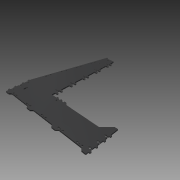
# Autodesk Inventor part: brace_right
Saved by Autodesk Inventor 2014 (Build 180170000, 170)
## iProperties
Created: 2013-12-03
Part Number: brace_right
Material: Generic
Document SubType Name: Modeling
Designer: buben
Density: 1 g/cm^3
Appearance: Anodized - Dark Gray
Author: buben
Subject: Laser Cutted
Autodesk Inventor part; units mm, degrees
ref_plane "YZ Plane" through (0, 0, 0) normal (1, 0, 0) x (0, 1, 0)
ref_plane "XZ Plane" through (0, 0, 0) normal (0, 1, 0) x (-1, 0, 0)
ref_plane "XY Plane" through (0, 0, 0) normal (0, 0, 1) x (1, 0, 0)
sketch "Sketch1" plane through (0, 0, 0) normal (0, 0, 1) x (1, 0, 0)
  line L0 (0, 0) -> (489, 0)
  line L1 (489, 0) -> (489, 150)
  line L2 (0, 0) -> (0, 120)
  line L3 (0, 120) -> (106.25, 518.5)
  line L4 (106.25, 518.5) -> (156.25, 518.5)
  line L5 (156.25, 518.5) -> (156.25, 113.5)
  line L6 (489, 150) -> (474, 150)
  line L7 (474, 150) -> (434, 110)
  line L8 (434, 110) -> (253.25, 110)
  line L9 (253.25, 110) -> (243.25, 120)
  line L10 (243.25, 120) -> (233.25, 120)
  line L11 (233.25, 120) -> (233.25, 113.5)
  line L12 (233.25, 113.5) -> (156.25, 113.5)
  point P0 (244.5, 0)
  dimension "d0" = 489
  dimension "d2" = 120
  dimension "d3" = 45
  dimension "d5" = 6.5
  dimension "d6" = 77
  dimension "d7" = 15
  dimension "d8" = 10
  dimension "d9" = 50
  dimension "d10" = 518.5
  dimension "d13" = 10
  dimension "d261" = 156.25
  dimension "d289" = 150
  dimension "d290" = 40
  constraints: 26 end point, 7 perpendicular, 3 parallel, 1 horizontal, 1 midpoint
  measures "d0" distance of L0.start L0.end
  measures "d2" distance of L0.start L2.end
  measures "d3" angle of L6 L7
  measures "d5" distance of L10.end L11.end
  measures "d6" distance of L11.end L5.end
  measures "d7" distance of L1.end L6.end
  measures "d8" distance of L9.end L10.end
  measures "d9" distance of L3.end L4.end
  measures "d10" distance between parallel lines of L0 L4
  measures "d13" distance between parallel lines of L8 L10
  measures "d261" distance between parallel lines of L2 L5
  measures "d289" distance of L0.end L1.end
  measures "d290" distance between parallel lines of L6 L8
extrude "Extrusion1" add sketch "Sketch1" along normal blind 6.5
sketch "Sketch2" plane through (0, 0, 6.5) normal (0, 0, 1) x (1, 0, 0)
  line L0 (0, 0) -> (489, 0) projected
  line L1 (489, 0) -> (489, 150) projected
  line L2 (253.25, 110) -> (243.25, 120) projected
  line L3 (489, 20.75) -> (489, 16.25)
  line L4 (472.7, 16.25) -> (472.7, 20.75)
  line L5 (476.7, 23.25) -> (484, 23.25)
  line L6 (484, 13.75) -> (476.7, 13.75)
  line L7 (472.7, 20.75) -> (476.7, 20.75)
  line L8 (484, 20.75) -> (489, 20.75)
  line L9 (489, 16.25) -> (484, 16.25)
  line L10 (476.7, 16.25) -> (472.7, 16.25)
  line L11 (476.7, 13.75) -> (476.7, 16.25)
  line L12 (476.7, 20.75) -> (476.7, 23.25)
  line L13 (484, 23.25) -> (484, 20.75)
  line L14 (484, 16.25) -> (484, 13.75)
  line L15 (489, 98.75) -> (489, 94.25)
  line L16 (472.7, 94.25) -> (472.7, 98.75)
  line L17 (476.7, 101.25) -> (484, 101.25)
  line L18 (484, 91.75) -> (476.7, 91.75)
  line L19 (472.7, 98.75) -> (476.7, 98.75)
  line L20 (484, 98.75) -> (489, 98.75)
  line L21 (489, 94.25) -> (484, 94.25)
  line L22 (476.7, 94.25) -> (472.7, 94.25)
  line L23 (476.7, 91.75) -> (476.7, 94.25)
  line L24 (476.7, 98.75) -> (476.7, 101.25)
  line L25 (484, 101.25) -> (484, 98.75)
  line L26 (484, 94.25) -> (484, 91.75)
  line L27 (489, 59.75) -> (489, 55.25)
  line L28 (472.7, 55.25) -> (472.7, 59.75)
  line L29 (476.7, 62.25) -> (484, 62.25)
  line L30 (484, 52.75) -> (476.7, 52.75)
  line L31 (472.7, 59.75) -> (476.7, 59.75)
  line L32 (484, 59.75) -> (489, 59.75)
  line L33 (489, 55.25) -> (484, 55.25)
  line L34 (476.7, 55.25) -> (472.7, 55.25)
  line L35 (476.7, 52.75) -> (476.7, 55.25)
  line L36 (476.7, 59.75) -> (476.7, 62.25)
  line L37 (484, 62.25) -> (484, 59.75)
  line L38 (484, 55.25) -> (484, 52.75)
  line L39 (244.5, 0) -> (244.5, 118.75) construction
  line L40 (0, 20.75) -> (0, 16.25)
  line L41 (16.3, 16.25) -> (16.3, 20.75)
  line L42 (12.3, 23.25) -> (5, 23.25)
  line L43 (5, 13.75) -> (12.3, 13.75)
  line L44 (16.3, 20.75) -> (12.3, 20.75)
  line L45 (5, 20.75) -> (0, 20.75)
  line L46 (0, 16.25) -> (5, 16.25)
  line L47 (12.3, 16.25) -> (16.3, 16.25)
  line L48 (12.3, 13.75) -> (12.3, 16.25)
  line L49 (12.3, 20.75) -> (12.3, 23.25)
  line L50 (5, 23.25) -> (5, 20.75)
  line L51 (5, 16.25) -> (5, 13.75)
  line L52 (16.3, 98.75) -> (12.3, 98.75)
  line L53 (16.3, 94.25) -> (16.3, 98.75)
  line L54 (12.3, 94.25) -> (16.3, 94.25)
  line L55 (12.3, 98.75) -> (12.3, 101.25)
  line L56 (12.3, 91.75) -> (12.3, 94.25)
  line L57 (12.3, 101.25) -> (5, 101.25)
  line L58 (5, 94.25) -> (5, 91.75)
  line L59 (5, 91.75) -> (12.3, 91.75)
  line L60 (5, 98.75) -> (0, 98.75)
  line L61 (0, 98.75) -> (0, 94.25)
  line L62 (0, 94.25) -> (5, 94.25)
  line L63 (5, 101.25) -> (5, 98.75)
  line L64 (12.3, 59.75) -> (12.3, 62.25)
  line L65 (16.3, 59.75) -> (12.3, 59.75)
  line L66 (16.3, 55.25) -> (16.3, 59.75)
  line L67 (12.3, 55.25) -> (16.3, 55.25)
  line L68 (12.3, 52.75) -> (12.3, 55.25)
  line L69 (12.3, 62.25) -> (5, 62.25)
  line L70 (5, 52.75) -> (12.3, 52.75)
  line L71 (5, 55.25) -> (5, 52.75)
  line L72 (5, 62.25) -> (5, 59.75)
  line L73 (0, 55.25) -> (5, 55.25)
  line L74 (5, 59.75) -> (0, 59.75)
  line L75 (0, 59.75) -> (0, 55.25)
  point P0 (472.7, 18.5)
  point P1 (480.35, 23.25)
  point P2 (472.7, 96.5)
  point P3 (480.35, 101.25)
  point P4 (472.7, 57.5)
  point P5 (480.35, 62.25)
  point P6 (16.3, 18.5)
  point P7 (8.65, 23.25)
  point P8 (16.3, 96.5)
  point P9 (8.65, 101.25)
  point P10 (16.3, 57.5)
  point P11 (8.65, 62.25)
  dimension "d16" = 4.5
  dimension "d17" = 2.5
  dimension "d18" = 2.5
  dimension "d19" = 4
  dimension "d20" = 7.3
  dimension "d21" = 5
  dimension "d23" = 4.5
  dimension "d24" = 2.5
  dimension "d25" = 2.5
  dimension "d26" = 4
  dimension "d27" = 7.3
  dimension "d28" = 5
  dimension "d30" = 4.5
  dimension "d31" = 2.5
  dimension "d32" = 2.5
  dimension "d33" = 4
  dimension "d34" = 7.3
  dimension "d35" = 5
  dimension "d40" = 18.5
  dimension "d41" = 39
  dimension "d42" = 39
  constraints: 146 end point, 42 symmetric about line, 30 parallel, 15 collinear, 13 perpendicular, 9 horizontal, 7 midpoint, 1 point on line
  measures "d16" distance of L4.start L4.end
  measures "d17" distance of L7.end L5.start
  measures "d18" distance of L6.end L10.start
  measures "d19" distance of L10.start L4.start
  measures "d20" distance of L6.start L6.end
  measures "d21" distance of L3.end L9.end
  measures "d23" distance of L16.start L19.start
  measures "d24" distance of L19.end L24.end
  measures "d25" distance of L23.start L22.start
  measures "d26" distance of L22.start L16.start
  measures "d27" distance of L26.end L23.start
  measures "d28" distance of L15.end L26.start
  measures "d30" distance of L28.start L31.start
  measures "d31" distance of L36.start L36.end
  measures "d32" distance of L35.start L34.start
  measures "d33" distance of L34.start L28.start
  measures "d34" distance of L30.start L35.start
  measures "d35" distance of L33.start L38.start
  measures "d40" distance from line of L0 point (472.7, 18.5)
  measures "d41" distance of point (472.7, 57.5) point (472.7, 18.5)
  measures "d42" distance of point (472.7, 57.5) point (472.7, 96.5)
extrude "Extrusion2" cut sketch "Sketch2" against normal through all
sketch "Sketch4" plane through (0, 0, 6.5) normal (0, 0, 1) x (1, 0, 0)
  line L0 (0, 16.25) -> (0, 0) projected
  line L1 (489, 0) -> (489, 16.25) projected
  line L2 (472.7, 16.25) -> (472.7, 20.75) projected
  line L3 (489, 20.75) -> (489, 55.25) projected
  line L4 (472.7, 55.25) -> (472.7, 59.75) projected
  line L5 (489, 59.75) -> (489, 94.25) projected
  line L6 (472.7, 94.25) -> (472.7, 98.75) projected
  line L7 (489, 98.75) -> (489, 150) projected
  line L8 (0, 120) -> (0, 98.75) projected
  line L9 (0, 94.25) -> (0, 59.75) projected
  line L10 (0, 55.25) -> (0, 20.75) projected
  line L11 (0, 112) -> (-4.5, 112)
  line L12 (-6.5, 110) -> (-6.5, 106)
  line L13 (-4.5, 104) -> (0, 104)
  line L14 (0, 104) -> (0, 112)
  line L15 (0, 81) -> (-4.5, 81)
  line L16 (-6.5, 79) -> (-6.5, 75)
  line L17 (-4.5, 73) -> (0, 73)
  line L18 (0, 73) -> (0, 81)
  line L19 (0, 42) -> (-4.5, 42)
  line L20 (-6.5, 40) -> (-6.5, 36)
  line L21 (-4.5, 34) -> (0, 34)
  line L22 (0, 34) -> (0, 42)
  line L23 (0, 11) -> (-4.5, 11)
  line L24 (-6.5, 9) -> (-6.5, 5)
  line L25 (-4.5, 3) -> (0, 3)
  line L26 (0, 3) -> (0, 11)
  line L27 (489, 112) -> (493.5, 112)
  line L28 (495.5, 110) -> (495.5, 106)
  line L29 (493.5, 104) -> (489, 104)
  line L30 (489, 104) -> (489, 112)
  line L31 (489, 81) -> (493.5, 81)
  line L32 (495.5, 79) -> (495.5, 75)
  line L33 (493.5, 73) -> (489, 73)
  line L34 (489, 73) -> (489, 81)
  line L35 (489, 42) -> (493.5, 42)
  line L36 (495.5, 40) -> (495.5, 36)
  line L37 (493.5, 34) -> (489, 34)
  line L38 (489, 34) -> (489, 42)
  line L39 (489, 11) -> (493.5, 11)
  line L40 (495.5, 9) -> (495.5, 5)
  line L41 (493.5, 3) -> (489, 3)
  line L42 (489, 3) -> (489, 11)
  arc A0 (-6.5, 5) -> (-4.5, 3) centre (-4.5, 5) ccw
  arc A1 (-4.5, 11) -> (-6.5, 9) centre (-4.5, 9) ccw
  arc A2 (-6.5, 36) -> (-4.5, 34) centre (-4.5, 36) ccw
  arc A3 (-4.5, 42) -> (-6.5, 40) centre (-4.5, 40) ccw
  arc A4 (-6.5, 75) -> (-4.5, 73) centre (-4.5, 75) ccw
  arc A5 (-4.5, 81) -> (-6.5, 79) centre (-4.5, 79) ccw
  arc A6 (-6.5, 106) -> (-4.5, 104) centre (-4.5, 106) ccw
  arc A7 (-4.5, 112) -> (-6.5, 110) centre (-4.5, 110) ccw
  arc A8 (495.5, 110) -> (493.5, 112) centre (493.5, 110) ccw
  arc A9 (493.5, 104) -> (495.5, 106) centre (493.5, 106) ccw
  arc A10 (495.5, 79) -> (493.5, 81) centre (493.5, 79) ccw
  arc A11 (493.5, 73) -> (495.5, 75) centre (493.5, 75) ccw
  arc A12 (495.5, 40) -> (493.5, 42) centre (493.5, 40) ccw
  arc A13 (493.5, 34) -> (495.5, 36) centre (493.5, 36) ccw
  arc A14 (495.5, 9) -> (493.5, 11) centre (493.5, 9) ccw
  arc A15 (493.5, 3) -> (495.5, 5) centre (493.5, 5) ccw
  line L43 (489, 20.75) -> (489, 55.25) projected
  point P0 (472.7, 96.5)
  point P1 (472.7, 57.5)
  point P2 (472.7, 18.5)
  point P3 (495.5, 77)
  point P4 (489, 77)
  point P5 (495.5, 38)
  point P6 (489, 38)
  dimension "d81" = 2
  dimension "d82" = 8
  dimension "d83" = 8
  dimension "d84" = 8
  dimension "d85" = 8
  dimension "d86" = 7.5
  dimension "d87" = 7.5
  dimension "d88" = 6.5
  dimension "d89" = 6.5
  constraints: 64 end point, 32 point on circle, 32 tangent, 16 centre point, 16 parallel, 15 equal radius, 14 collinear, 8 horizontal, 8 perpendicular, 8 point on line, 7 midpoint, 2 horizontal alignment
  measures "d81" radius of A0
  measures "d82" distance between parallel lines of L29 L27
  measures "d83" distance between parallel lines of L33 L31
  measures "d84" distance between parallel lines of L37 L35
  measures "d85" distance between parallel lines of L41 L39
  measures "d86" distance from line of point (472.7, 96.5) L29
  measures "d87" distance from line of point (472.7, 18.5) L39
  measures "d88" distance between parallel lines of L7 L28
  measures "d89" distance between parallel lines of L8 L12
extrude "Extrusion4" add sketch "Sketch4" against normal blind 6.5
sketch "Sketch5" plane through (0, 0, 6.5) normal (0, 0, 1) x (1, 0, 0)
  line L0 (233.25, 120) -> (233.25, 113.5) projected
  line L1 (233.25, 113.5) -> (156.25, 113.5) projected
  line L2 (201.5, 113.5) -> (206, 113.5)
  line L3 (206, 97.2) -> (201.5, 97.2)
  line L4 (208.5, 108.5) -> (208.5, 101.2)
  line L5 (199, 101.2) -> (199, 108.5)
  line L6 (206, 113.5) -> (206, 108.5)
  line L7 (206, 101.2) -> (206, 97.2)
  line L8 (201.5, 97.2) -> (201.5, 101.2)
  line L9 (201.5, 108.5) -> (201.5, 113.5)
  line L10 (199, 108.5) -> (201.5, 108.5)
  line L11 (206, 108.5) -> (208.5, 108.5)
  line L12 (208.5, 101.2) -> (206, 101.2)
  line L13 (201.5, 101.2) -> (199, 101.2)
  point P0 (203.75, 97.2)
  dimension "d92" = 4.5
  dimension "d93" = 2.5
  dimension "d94" = 2.5
  dimension "d95" = 5
  dimension "d96" = 7.3
  dimension "d97" = 4
  dimension "d98" = 29.5
  constraints: 24 end point, 10 parallel, 5 collinear, 4 perpendicular, 3 horizontal, 1 midpoint
  measures "d92" distance of L3.start L3.end
  measures "d93" distance of L8.end L5.start
  measures "d94" distance of L4.end L7.start
  measures "d95" distance of L2.end L6.end
  measures "d96" distance of L4.start L4.end
  measures "d97" distance of L7.start L3.start
  measures "d98" distance from line of L0 point (203.75, 97.2)
extrude "Extrusion5" cut sketch "Sketch5" against normal through all
sketch "Sketch6" plane through (0, 0, 6.5) normal (0, 0, 1) x (1, 0, 0)
  line L0 (206, 97.2) -> (201.5, 97.2) projected
  line L1 (201.5, 113.5) -> (156.25, 113.5) projected
  line L2 (233.25, 113.5) -> (206, 113.5) projected
  line L3 (188.25, 113.5) -> (196.25, 113.5)
  line L4 (196.25, 113.5) -> (196.25, 118)
  line L5 (194.25, 120) -> (190.25, 120)
  line L6 (188.25, 118) -> (188.25, 113.5)
  line L7 (211.25, 113.5) -> (219.25, 113.5)
  line L8 (219.25, 113.5) -> (219.25, 118)
  line L9 (217.25, 120) -> (213.25, 120)
  line L10 (211.25, 118) -> (211.25, 113.5)
  arc A0 (190.25, 120) -> (188.25, 118) centre (190.25, 118) ccw
  arc A1 (196.25, 118) -> (194.25, 120) centre (194.25, 118) ccw
  arc A2 (213.25, 120) -> (211.25, 118) centre (213.25, 118) ccw
  arc A3 (219.25, 118) -> (217.25, 120) centre (217.25, 118) ccw
  point P0 (203.75, 97.2)
  dimension "d101" = 2
  dimension "d102" = 15
  dimension "d103" = 8
  dimension "d104" = 8
  dimension "d105" = 7.5
  dimension "d106" = 6.5
  constraints: 16 end point, 8 point on circle, 8 tangent, 4 centre point, 4 parallel, 3 equal radius, 2 horizontal, 2 perpendicular, 2 point on line, 1 collinear, 1 midpoint
  measures "d101" radius of A0
  measures "d102" distance between parallel lines of L4 L10
  measures "d103" distance between parallel lines of L6 L4
  measures "d104" distance between parallel lines of L8 L10
  measures "d105" distance from line of point (203.75, 97.2) L4
  measures "d106" distance between parallel lines of L1 L5
extrude "Extrusion6" add sketch "Sketch6" against normal blind 6.5
sketch "Sketch7" plane through (0, 0, 6.5) normal (0, 0, 1) x (1, 0, 0)
  line L0 (156.25, 113.5) -> (156.25, 518.5) projected
  line L1 (156.25, 518.5) -> (106.25, 518.5) projected
  line L2 (121.25, 451) -> (113.25, 451)
  line L3 (113.25, 451) -> (113.25, 444.5)
  line L4 (113.25, 444.5) -> (121.25, 444.5)
  line L5 (121.25, 444.5) -> (121.25, 451)
  circle A0 centre (128.75, 447.75) radius 2.25
  point P0 (121.25, 447.75)
  dimension "d109" = 6.5
  dimension "d110" = 8
  dimension "d118" = 7.5
  dimension "d119" = 27.5
  dimension "d121" = 4.5
  dimension "d288" = 74
  constraints: 8 end point, 2 parallel, 1 centre point, 1 horizontal, 1 horizontal alignment, 1 midpoint, 1 perpendicular
  measures "d109" distance of L2.end L3.end
  measures "d110" distance of L2.start L2.end
  measures "d118" distance from line of A0.centre L5
  measures "d119" distance from line of L0 A0.centre
  measures "d121" diameter of A0
  measures "d288" distance between parallel lines of L4 L1
extrude "Extrusion8" cut sketch "Sketch7" against normal through all
sketch "Sketch8" plane through (0, 0, 6.5) normal (0, 0, 1) x (1, 0, 0)
  line L0 (156.25, 518.5) -> (112.25, 518.5)
  line L1 (112.25, 518.5) -> (112.25, 512)
  line L2 (112.25, 512) -> (156.25, 512)
  line L3 (156.25, 512) -> (156.25, 518.5)
  point P0 (106.25, 518.5)
  dimension "d124" = 6
  dimension "d125" = 6.5
  constraints: 8 end point, 2 parallel, 1 horizontal, 1 perpendicular
  measures "d124" distance from line of point (106.25, 518.5) L1
  measures "d125" distance of L0.end L1.end
extrude "Extrusion9" cut sketch "Sketch8" against normal through all
sketch "Sketch9" plane through (0, 0, 6.5) normal (0, 0, 1) x (1, 0, 0)
  line L0 (156.25, 113.5) -> (156.25, 512) projected
  line L1 (156.25, 470.75) -> (156.25, 466.25)
  line L2 (139.95, 466.25) -> (139.95, 470.75)
  line L3 (143.95, 473.25) -> (151.25, 473.25)
  line L4 (151.25, 463.75) -> (143.95, 463.75)
  line L5 (151.25, 473.25) -> (151.25, 470.75)
  line L6 (151.25, 466.25) -> (151.25, 463.75)
  line L7 (143.95, 463.75) -> (143.95, 466.25)
  line L8 (143.95, 470.75) -> (143.95, 473.25)
  line L9 (139.95, 470.75) -> (143.95, 470.75)
  line L10 (151.25, 470.75) -> (156.25, 470.75)
  line L11 (156.25, 466.25) -> (151.25, 466.25)
  line L12 (143.95, 466.25) -> (139.95, 466.25)
  line L13 (156.25, 390.75) -> (156.25, 386.25)
  line L14 (139.95, 386.25) -> (139.95, 390.75)
  line L15 (143.95, 393.25) -> (151.25, 393.25)
  line L16 (151.25, 383.75) -> (143.95, 383.75)
  line L17 (151.25, 393.25) -> (151.25, 390.75)
  line L18 (151.25, 386.25) -> (151.25, 383.75)
  line L19 (143.95, 383.75) -> (143.95, 386.25)
  line L20 (143.95, 390.75) -> (143.95, 393.25)
  line L21 (139.95, 390.75) -> (143.95, 390.75)
  line L22 (151.25, 390.75) -> (156.25, 390.75)
  line L23 (156.25, 386.25) -> (151.25, 386.25)
  line L24 (143.95, 386.25) -> (139.95, 386.25)
  line L25 (156.25, 310.75) -> (156.25, 306.25)
  line L26 (139.95, 306.25) -> (139.95, 310.75)
  line L27 (143.95, 313.25) -> (151.25, 313.25)
  line L28 (151.25, 303.75) -> (143.95, 303.75)
  line L29 (151.25, 313.25) -> (151.25, 310.75)
  line L30 (151.25, 306.25) -> (151.25, 303.75)
  line L31 (143.95, 303.75) -> (143.95, 306.25)
  line L32 (143.95, 310.75) -> (143.95, 313.25)
  line L33 (139.95, 310.75) -> (143.95, 310.75)
  line L34 (151.25, 310.75) -> (156.25, 310.75)
  line L35 (156.25, 306.25) -> (151.25, 306.25)
  line L36 (143.95, 306.25) -> (139.95, 306.25)
  line L37 (156.25, 230.75) -> (156.25, 226.25)
  line L38 (139.95, 226.25) -> (139.95, 230.75)
  line L39 (143.95, 233.25) -> (151.25, 233.25)
  line L40 (151.25, 223.75) -> (143.95, 223.75)
  line L41 (151.25, 233.25) -> (151.25, 230.75)
  line L42 (151.25, 226.25) -> (151.25, 223.75)
  line L43 (143.95, 223.75) -> (143.95, 226.25)
  line L44 (143.95, 230.75) -> (143.95, 233.25)
  line L45 (139.95, 230.75) -> (143.95, 230.75)
  line L46 (151.25, 230.75) -> (156.25, 230.75)
  line L47 (156.25, 226.25) -> (151.25, 226.25)
  line L48 (143.95, 226.25) -> (139.95, 226.25)
  line L49 (156.25, 150.75) -> (156.25, 146.25)
  line L50 (139.95, 146.25) -> (139.95, 150.75)
  line L51 (143.95, 153.25) -> (151.25, 153.25)
  line L52 (151.25, 143.75) -> (143.95, 143.75)
  line L53 (151.25, 153.25) -> (151.25, 150.75)
  line L54 (151.25, 146.25) -> (151.25, 143.75)
  line L55 (143.95, 143.75) -> (143.95, 146.25)
  line L56 (143.95, 150.75) -> (143.95, 153.25)
  line L57 (139.95, 150.75) -> (143.95, 150.75)
  line L58 (151.25, 150.75) -> (156.25, 150.75)
  line L59 (156.25, 146.25) -> (151.25, 146.25)
  line L60 (143.95, 146.25) -> (139.95, 146.25)
  line L61 (112.25, 518.5) -> (106.25, 518.5) projected
  point P0 (139.95, 468.5)
  point P1 (139.95, 388.5)
  point P2 (139.95, 308.5)
  point P3 (139.95, 228.5)
  point P4 (139.95, 148.5)
  dimension "d128" = 4.5
  dimension "d129" = 2.5
  dimension "d130" = 2.5
  dimension "d131" = 5
  dimension "d132" = 7.3
  dimension "d133" = 4
  dimension "d137" = 80
  dimension "d286" = 50
  constraints: 120 end point, 10 parallel, 5 collinear, 4 perpendicular, 3 horizontal, 1 midpoint, 1 vertical, 100 other
  measures "d128" distance of L2.start L2.end
  measures "d129" distance of L8.start L3.start
  measures "d130" distance of L4.end L7.end
  measures "d131" distance of L1.end L6.start
  measures "d132" distance of L4.start L4.end
  measures "d133" distance of L7.end L2.start
  measures "d137" distance of L1.end L23.start
  measures "d286" distance from line of L61 point (139.95, 468.5)
extrude "Extrusion10" cut sketch "Sketch9" against normal through all
sketch "Sketch10" plane through (0, 0, 6.5) normal (0, 0, 1) x (1, 0, 0)
  line L0 (156.25, 390.75) -> (156.25, 466.25) projected
  line L1 (139.95, 466.25) -> (139.95, 470.75) projected
  line L2 (156.25, 470.75) -> (156.25, 512) projected
  line L3 (156.25, 484) -> (167.25, 484)
  line L4 (169.25, 482) -> (169.25, 478)
  line L5 (167.25, 476) -> (156.25, 476)
  line L6 (156.25, 476) -> (156.25, 484)
  line L7 (156.25, 461) -> (167.25, 461)
  line L8 (169.25, 459) -> (169.25, 455)
  line L9 (167.25, 453) -> (156.25, 453)
  line L10 (156.25, 453) -> (156.25, 461)
  arc A0 (169.25, 482) -> (167.25, 484) centre (167.25, 482) ccw
  arc A1 (167.25, 476) -> (169.25, 478) centre (167.25, 478) ccw
  arc A2 (169.25, 459) -> (167.25, 461) centre (167.25, 459) ccw
  arc A3 (167.25, 453) -> (169.25, 455) centre (167.25, 455) ccw
  line L11 (156.25, 404) -> (167.25, 404)
  line L12 (169.25, 402) -> (169.25, 398)
  line L13 (167.25, 396) -> (156.25, 396)
  line L14 (156.25, 396) -> (156.25, 404)
  line L15 (156.25, 381) -> (167.25, 381)
  line L16 (169.25, 379) -> (169.25, 375)
  line L17 (167.25, 373) -> (156.25, 373)
  line L18 (156.25, 373) -> (156.25, 381)
  arc A4 (169.25, 402) -> (167.25, 404) centre (167.25, 402) ccw
  arc A5 (167.25, 396) -> (169.25, 398) centre (167.25, 398) ccw
  arc A6 (169.25, 379) -> (167.25, 381) centre (167.25, 379) ccw
  arc A7 (167.25, 373) -> (169.25, 375) centre (167.25, 375) ccw
  line L19 (156.25, 324) -> (167.25, 324)
  line L20 (169.25, 322) -> (169.25, 318)
  line L21 (167.25, 316) -> (156.25, 316)
  line L22 (156.25, 316) -> (156.25, 324)
  line L23 (156.25, 301) -> (167.25, 301)
  line L24 (169.25, 299) -> (169.25, 295)
  line L25 (167.25, 293) -> (156.25, 293)
  line L26 (156.25, 293) -> (156.25, 301)
  arc A8 (169.25, 322) -> (167.25, 324) centre (167.25, 322) ccw
  arc A9 (167.25, 316) -> (169.25, 318) centre (167.25, 318) ccw
  arc A10 (169.25, 299) -> (167.25, 301) centre (167.25, 299) ccw
  arc A11 (167.25, 293) -> (169.25, 295) centre (167.25, 295) ccw
  line L27 (156.25, 244) -> (167.25, 244)
  line L28 (169.25, 242) -> (169.25, 238)
  line L29 (167.25, 236) -> (156.25, 236)
  line L30 (156.25, 236) -> (156.25, 244)
  line L31 (156.25, 221) -> (167.25, 221)
  line L32 (169.25, 219) -> (169.25, 215)
  line L33 (167.25, 213) -> (156.25, 213)
  line L34 (156.25, 213) -> (156.25, 221)
  arc A12 (169.25, 242) -> (167.25, 244) centre (167.25, 242) ccw
  arc A13 (167.25, 236) -> (169.25, 238) centre (167.25, 238) ccw
  arc A14 (169.25, 219) -> (167.25, 221) centre (167.25, 219) ccw
  arc A15 (167.25, 213) -> (169.25, 215) centre (167.25, 215) ccw
  line L35 (156.25, 164) -> (167.25, 164)
  line L36 (169.25, 162) -> (169.25, 158)
  line L37 (167.25, 156) -> (156.25, 156)
  line L38 (156.25, 156) -> (156.25, 164)
  line L39 (156.25, 141) -> (167.25, 141)
  line L40 (169.25, 139) -> (169.25, 135)
  line L41 (167.25, 133) -> (156.25, 133)
  line L42 (156.25, 133) -> (156.25, 141)
  arc A16 (169.25, 162) -> (167.25, 164) centre (167.25, 162) ccw
  arc A17 (167.25, 156) -> (169.25, 158) centre (167.25, 158) ccw
  arc A18 (169.25, 139) -> (167.25, 141) centre (167.25, 139) ccw
  arc A19 (167.25, 133) -> (169.25, 135) centre (167.25, 135) ccw
  point P0 (139.95, 468.5)
  dimension "d144" = 2
  dimension "d145" = 8
  dimension "d146" = 8
  dimension "d147" = 13
  dimension "d148" = 15
  dimension "d149" = 7.5
  dimension "d152" = 80
  constraints: 80 end point, 40 point on circle, 20 centre point, 8 tangent, 4 parallel, 3 equal radius, 2 horizontal, 2 perpendicular, 2 point on line, 1 collinear, 1 midpoint, 1 vertical, 112 other
  measures "d144" radius of A0
  measures "d145" distance between parallel lines of L9 L7
  measures "d146" distance between parallel lines of L5 L3
  measures "d147" distance between parallel lines of L6 L4
  measures "d148" distance between parallel lines of L5 L7
  measures "d149" distance from line of L5 point (139.95, 468.5)
  measures "d152" distance of A1.centre A5.centre
extrude "Extrusion11" add sketch "Sketch10" against normal blind 6.5
sketch "Sketch11" plane through (0, 0, 6.5) normal (0, 0, 1) x (1, 0, 0)
  line L0 (156.25, 512) -> (112.25, 512) projected
  line L1 (126.269, 512) -> (130.769, 512)
  line L2 (130.769, 495.7) -> (126.269, 495.7)
  line L3 (133.269, 507) -> (133.269, 499.7)
  line L4 (123.769, 499.7) -> (123.769, 507)
  line L5 (123.769, 507) -> (126.269, 507)
  line L6 (130.769, 507) -> (133.269, 507)
  line L7 (133.269, 499.7) -> (130.769, 499.7)
  line L8 (126.269, 499.7) -> (123.769, 499.7)
  line L9 (126.269, 495.7) -> (126.269, 499.7)
  line L10 (126.269, 507) -> (126.269, 512)
  line L11 (130.769, 512) -> (130.769, 507)
  line L12 (130.769, 499.7) -> (130.769, 495.7)
  line L13 (156.25, 484) -> (156.25, 512) projected
  point P0 (128.519, 495.7)
  dimension "d159" = 4.5
  dimension "d160" = 2.5
  dimension "d161" = 2.5
  dimension "d162" = 5
  dimension "d163" = 7.3
  dimension "d164" = 4
  dimension "d235" = 27.731
  constraints: 24 end point, 10 parallel, 5 collinear, 4 perpendicular, 3 horizontal, 1 midpoint
  measures "d159" distance of L2.start L2.end
  measures "d160" distance of L3.end L7.end
  measures "d161" distance of L8.start L4.start
  measures "d162" distance of L1.end L6.start
  measures "d163" distance of L3.start L3.end
  measures "d164" distance of L7.end L2.start
  measures "d235" distance from line of L13 point (128.519, 495.7)
extrude "Extrusion12" cut sketch "Sketch11" against normal through all
sketch "Sketch12" plane through (0, 0, 6.5) normal (0, 0, 1) x (1, 0, 0)
  line L0 (0, 0) -> (489, 0) projected
  line L1 (30, 9.5) -> (38, 9.5)
  line L2 (38, 9.5) -> (38, 3)
  line L3 (38, 3) -> (30, 3)
  line L4 (30, 3) -> (30, 9.5)
  line L5 (53, 9.5) -> (61, 9.5)
  line L6 (61, 9.5) -> (61, 3)
  line L7 (61, 3) -> (53, 3)
  line L8 (53, 3) -> (53, 9.5)
  line L9 (38, 9.5) -> (53, 3) construction
  line L10 (53, 9.5) -> (38, 3) construction
  circle A0 centre (45.5, 6.25) radius 2.25
  line L11 (129.5, 9.5) -> (137.5, 9.5)
  line L12 (137.5, 9.5) -> (137.5, 3)
  line L13 (137.5, 3) -> (129.5, 3)
  line L14 (129.5, 3) -> (129.5, 9.5)
  line L15 (152.5, 9.5) -> (160.5, 9.5)
  line L16 (160.5, 9.5) -> (160.5, 3)
  line L17 (160.5, 3) -> (152.5, 3)
  line L18 (152.5, 3) -> (152.5, 9.5)
  line L19 (137.5, 9.5) -> (152.5, 3) construction
  line L20 (152.5, 9.5) -> (137.5, 3) construction
  circle A1 centre (145, 6.25) radius 2.25
  line L21 (328.5, 9.5) -> (336.5, 9.5)
  line L22 (336.5, 9.5) -> (336.5, 3)
  line L23 (336.5, 3) -> (328.5, 3)
  line L24 (328.5, 3) -> (328.5, 9.5)
  line L25 (351.5, 9.5) -> (359.5, 9.5)
  line L26 (359.5, 9.5) -> (359.5, 3)
  line L27 (359.5, 3) -> (351.5, 3)
  line L28 (351.5, 3) -> (351.5, 9.5)
  line L29 (336.5, 9.5) -> (351.5, 3) construction
  line L30 (351.5, 9.5) -> (336.5, 3) construction
  circle A2 centre (344, 6.25) radius 2.25
  line L31 (428, 9.5) -> (436, 9.5)
  line L32 (436, 9.5) -> (436, 3)
  line L33 (436, 3) -> (428, 3)
  line L34 (428, 3) -> (428, 9.5)
  line L35 (451, 9.5) -> (459, 9.5)
  line L36 (459, 9.5) -> (459, 3)
  line L37 (459, 3) -> (451, 3)
  line L38 (451, 3) -> (451, 9.5)
  line L39 (436, 9.5) -> (451, 3) construction
  line L40 (451, 9.5) -> (436, 3) construction
  circle A3 centre (443.5, 6.25) radius 2.25
  line L41 (229, 9.5) -> (237, 9.5)
  line L42 (237, 9.5) -> (237, 3)
  line L43 (237, 3) -> (229, 3)
  line L44 (229, 3) -> (229, 9.5)
  line L45 (252, 9.5) -> (260, 9.5)
  line L46 (260, 9.5) -> (260, 3)
  line L47 (260, 3) -> (252, 3)
  line L48 (252, 3) -> (252, 9.5)
  line L49 (237, 9.5) -> (252, 3) construction
  line L50 (252, 9.5) -> (237, 3) construction
  circle A4 centre (244.5, 6.25) radius 2.25
  line L51 (61, 6.25) -> (129.5, 6.25) construction
  line L52 (160.5, 6.25) -> (229, 6.25) construction
  line L53 (260, 6.25) -> (328.5, 6.25) construction
  line L54 (359.5, 6.25) -> (428, 6.25) construction
  point P0 (145, 6.25)
  point P1 (344, 6.25)
  dimension "d168" = 8
  dimension "d169" = 8
  dimension "d170" = 6.5
  dimension "d171" = 15
  dimension "d172" = 4.5
  dimension "d173" = 8
  dimension "d174" = 8
  dimension "d175" = 6.5
  dimension "d176" = 15
  dimension "d177" = 4.5
  dimension "d178" = 8
  dimension "d179" = 8
  dimension "d180" = 6.5
  dimension "d181" = 15
  dimension "d182" = 4.5
  dimension "d183" = 8
  dimension "d184" = 8
  dimension "d185" = 6.5
  dimension "d186" = 15
  dimension "d187" = 4.5
  dimension "d188" = 8
  dimension "d189" = 8
  dimension "d190" = 6.5
  dimension "d191" = 15
  dimension "d192" = 4.5
  dimension "d198" = 3
  dimension "d206" = 30
  dimension "d207" = 30
  constraints: 108 end point, 20 parallel, 15 midpoint, 13 collinear, 10 horizontal, 10 perpendicular, 5 centre point, 4 horizontal alignment
  measures "d168" distance of L1.start L1.end
  measures "d169" distance of L5.start L5.end
  measures "d170" distance of L3.end L1.start
  measures "d171" distance between parallel lines of L8 L2
  measures "d172" diameter of A0
  measures "d173" distance of L11.start L11.end
  measures "d174" distance of L15.start L15.end
  measures "d175" distance of L14.start L11.start
  measures "d176" distance between parallel lines of L18 L12
  measures "d177" diameter of A1
  measures "d178" distance of L21.start L21.end
  measures "d179" distance of L25.start L25.end
  measures "d180" distance of L24.start L21.start
  measures "d181" distance between parallel lines of L28 L22
  measures "d182" diameter of A2
  measures "d183" distance of L31.start L31.end
  measures "d184" distance of L35.start L35.end
  measures "d185" distance of L34.start L31.start
  measures "d186" distance between parallel lines of L38 L32
  measures "d187" diameter of A3
  measures "d188" distance of L41.start L41.end
  measures "d189" distance of L45.start L45.end
  measures "d190" distance of L44.start L41.start
  measures "d191" distance between parallel lines of L48 L42
  measures "d192" diameter of A4
  measures "d198" distance between parallel lines of L0 L3
  measures "d206" distance from line of L0.end L36
  measures "d207" distance from line of L0.start L4
extrude "Extrusion13" cut sketch "Sketch12" against normal through all
sketch "Sketch13" plane through (0, 0, 6.5) normal (0, 0, 1) x (1, 0, 0)
  line L0 (0, 0) -> (489, 0) projected
  line L1 (121.25, 444.5) -> (113.25, 444.5) projected
  line L2 (0, 0) -> (0, -10)
  line L3 (0, -10) -> (20, -10)
  line L4 (20, -10) -> (30, 0)
  line L5 (146.3333, 0) -> (156.3333, -10)
  line L6 (156.3333, -10) -> (176.3333, -10)
  line L7 (176.3333, -10) -> (186.3333, 0)
  line L8 (302.6667, 0) -> (312.6667, -10)
  line L9 (312.6667, -10) -> (332.6667, -10)
  line L10 (332.6667, -10) -> (342.6667, 0)
  line L11 (489, 0) -> (489, -10)
  line L12 (489, -10) -> (469, -10)
  line L13 (469, -10) -> (459, 0)
  line L14 (20, -10) -> (156.3333, -10) construction
  line L15 (176.3333, -10) -> (312.6667, -10) construction
  line L16 (332.6667, -10) -> (469, -10) construction
  dimension "d201" = 10
  dimension "d202" = 20
  dimension "d203" = 45
  constraints: 30 end point, 13 collinear, 9 perpendicular, 6 point on line
  measures "d201" distance of L0.start L2.end
  measures "d202" distance of L2.end L3.end
  measures "d203" angle of L3 L4
extrude "Extrusion14" add sketch "Sketch13" against normal blind 6.5
sketch "Sketch14" plane through (0, 0, 6.5) normal (0, 0, 1) x (1, 0, 0)
  line L0 (252, 3) -> (252, 9.5) projected
  line L1 (0, 73) -> (0, 59.75) projected
  line L2 (30, 0) -> (146.3333, 0) projected
  line L3 (40, 69) -> (40, 54) construction
  line L4 (36, 69) -> (36, 54)
  line L5 (44, 54) -> (44, 69)
  arc A0 (44, 69) -> (36, 69) centre (40, 69) ccw
  arc A1 (36, 54) -> (44, 54) centre (40, 54) ccw
  point P0 (0, 0)
  point P1 (40, 61.5)
  dimension "d208" = 15
  dimension "d209" = 8
  dimension "d210" = 54
  dimension "d211" = 40
  constraints: 8 end point, 4 point on circle, 4 tangent, 2 centre point, 2 parallel, 1 midpoint
  measures "d208" distance of L3.start L3.end
  measures "d209" distance between parallel lines of L5 L4
  measures "d210" distance from line of L3.end L2
  measures "d211" distance between parallel lines of L1 L3
extrude "Extrusion15" cut sketch "Sketch14" against normal through all
sketch "Sketch19" plane through (0, 0, 6.5) normal (0, 0, 1) x (1, 0, 0)
  line L0 (106.25, 518.5) -> (0, 120) projected
  line L1 (107.1853, 510.363) -> (113.4659, 508.6884) construction
  line L2 (113.4659, 508.6884) -> (9.3854, 118.3254) construction
  line L3 (9.3854, 118.3254) -> (3.1048, 120) construction
  line L4 (3.1048, 120) -> (107.1853, 510.363) construction
  circle A0 centre (27.0612, 197.2353) radius 2.25
  circle A1 centre (47.8773, 275.3079) radius 2.25
  circle A2 centre (68.6934, 353.3805) radius 2.25
  circle A3 centre (89.5095, 431.4531) radius 2.25
  line L5 (6.2451, 119.1627) -> (27.0612, 197.2353) construction
  line L6 (27.0612, 197.2353) -> (47.8773, 275.3079) construction
  line L7 (47.8773, 275.3079) -> (68.6934, 353.3805) construction
  line L8 (68.6934, 353.3805) -> (89.5095, 431.4531) construction
  line L9 (89.5095, 431.4531) -> (110.3256, 509.5257) construction
  line L10 (21.9887, 190.8258) -> (28.2693, 189.1512)
  line L11 (28.2693, 189.1512) -> (26.2083, 181.4212)
  line L12 (26.2083, 181.4212) -> (19.9277, 183.0958)
  line L13 (19.9277, 183.0958) -> (21.9887, 190.8258)
  line L14 (27.9141, 213.0494) -> (34.1947, 211.3748)
  line L15 (34.1947, 211.3748) -> (32.1337, 203.6449)
  line L16 (32.1337, 203.6449) -> (25.8531, 205.3194)
  line L17 (25.8531, 205.3194) -> (27.9141, 213.0494)
  line L18 (48.7302, 291.122) -> (55.0108, 289.4474)
  line L19 (55.0108, 289.4474) -> (52.9498, 281.7175)
  line L20 (52.9498, 281.7175) -> (46.6692, 283.392)
  line L21 (46.6692, 283.392) -> (48.7302, 291.122)
  line L22 (42.8048, 268.8984) -> (49.0854, 267.2238)
  line L23 (49.0854, 267.2238) -> (47.0244, 259.4938)
  line L24 (47.0244, 259.4938) -> (40.7438, 261.1684)
  line L25 (40.7438, 261.1684) -> (42.8048, 268.8984)
  line L26 (69.5463, 369.1946) -> (75.8269, 367.52)
  line L27 (75.8269, 367.52) -> (73.7659, 359.7901)
  line L28 (73.7659, 359.7901) -> (67.4853, 361.4646)
  line L29 (67.4853, 361.4646) -> (69.5463, 369.1946)
  line L30 (63.6209, 346.971) -> (69.9015, 345.2964)
  line L31 (69.9015, 345.2964) -> (67.8405, 337.5664)
  line L32 (67.8405, 337.5664) -> (61.5599, 339.241)
  line L33 (61.5599, 339.241) -> (63.6209, 346.971)
  line L34 (90.3624, 447.2672) -> (96.643, 445.5926)
  line L35 (96.643, 445.5926) -> (94.582, 437.8627)
  line L36 (94.582, 437.8627) -> (88.3014, 439.5372)
  line L37 (88.3014, 439.5372) -> (90.3624, 447.2672)
  line L38 (84.437, 425.0435) -> (90.7176, 423.369)
  line L39 (90.7176, 423.369) -> (88.6566, 415.639)
  line L40 (88.6566, 415.639) -> (82.376, 417.3136)
  line L41 (82.376, 417.3136) -> (84.437, 425.0435)
  line L42 (121.25, 444.5) -> (113.25, 444.5) projected
  line L43 (113.4659, 508.6884) -> (116.0819, 518.5)
  line L44 (156.25, 512) -> (156.25, 518.5)
  point P0 (0, 0)
  point P1 (112.25, 518.5)
  dimension "d262" = 6.5
  dimension "d263" = 3
  dimension "d266" = 3.25
  dimension "d267" = 3.25
  dimension "d268" = 3.25
  dimension "d269" = 3.25
  dimension "d270" = 4.5
  dimension "d271" = 404
  dimension "d274" = 8
  dimension "d275" = 15
  dimension "d276" = 15
  dimension "d277" = 15
  dimension "d279" = 15
  dimension "d280" = 7.5
  dimension "d281" = 7.5
  dimension "d282" = 7.5
  dimension "d283" = 7.5
  constraints: 86 end point, 18 collinear, 18 parallel, 11 equal length, 11 perpendicular, 4 centre point, 3 equal radius, 3 horizontal alignment, 2 midpoint
  measures "d262" distance between parallel lines of L4 L2
  measures "d263" distance between parallel lines of L0 L4
  measures "d266" distance from line of L2 L5.end
  measures "d267" distance from line of L2 L6.end
  measures "d268" distance from line of L2 L7.end
  measures "d269" distance from line of L2 L8.end
  measures "d270" diameter of A0
  measures "d271" distance of L1.end L2.end
  measures "d274" distance of L12.end L10.start
  measures "d275" distance between parallel lines of L16 L10
  measures "d276" distance between parallel lines of L20 L22
  measures "d277" distance between parallel lines of L28 L30
  measures "d279" distance between parallel lines of L36 L38
  measures "d280" distance from line of L5.end L10
  measures "d281" distance from line of L6.end L22
  measures "d282" distance from line of L7.end L30
  measures "d283" distance from line of L8.end L38
extrude "Extrusion20" cut sketch "Sketch19" against normal through all
body "Solid1"
